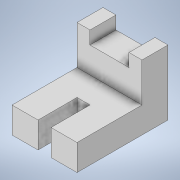
# Autodesk Inventor part: 4.2 Part C
Saved by Autodesk Inventor 2020 (Build 240168000, 168)
## iProperties
Created: 2020-01-07
Part Number: 4.2 Part C
Material: Generic
Document SubType Name: Modeling
Designer: cks4a449
Density: 1 g/cm^3
Appearance: Default
Author: cks4a449
Autodesk Inventor part; units mm, degrees
ref_plane "YZ Plane" through (0, 0, 0) normal (1, 0, 0) x (0, 1, 0)
ref_plane "XZ Plane" through (0, 0, 0) normal (0, 1, 0) x (-1, 0, 0)
ref_plane "XY Plane" through (0, 0, 0) normal (0, 0, 1) x (1, 0, 0)
sketch "Sketch1" plane through (0, 0, 0) normal (0, 0, 1) x (1, 0, 0)
  line L0 (0, 0) -> (88.9, 0)
  line L1 (88.9, 0) -> (88.9, 63.5)
  line L2 (88.9, 63.5) -> (63.5, 63.5)
  line L3 (63.5, 63.5) -> (63.5, 25.4)
  line L4 (63.5, 25.4) -> (0, 25.4)
  line L5 (0, 25.4) -> (0, 0)
  dimension "d0" = 88.9
  dimension "d1" = 63.5
  dimension "d2" = 25.4
  dimension "d3" = 38.1
  constraints: 12 end point, 5 perpendicular, 1 horizontal
  measures "d0" distance of L0.start L0.end
  measures "d1" distance of L0.end L1.end
  measures "d2" distance of L1.end L2.end
  measures "d3" distance of L2.end L3.end
extrude "Extrusion1" add sketch "Sketch1" along normal blind 63.5
sketch "Sketch2" plane through (63.5, 63.5, 0) normal (0, 1, 0) x (1, 0, 0)
  line L0 (25.4, 0) -> (25.4, -63.5) projected
  line L1 (25.4, 0) -> (0, 0)
  line L2 (0, 0) -> (0, -12.7)
  line L3 (0, -12.7) -> (25.4, -12.7)
  line L4 (25.4, -12.7) -> (25.4, 0)
  line L5 (25.4, -12.7) -> (0, -12.7)
  line L6 (0, -12.7) -> (0, -50.8)
  line L7 (0, -50.8) -> (25.4, -50.8)
  line L8 (25.4, -50.8) -> (25.4, -12.7)
  point P0 (-63.5, 0)
  dimension "d6" = 25.4
  dimension "d7" = 12.7
  dimension "d8" = 25.4
  dimension "d9" = 38.1
  constraints: 16 end point, 4 parallel, 2 horizontal, 2 perpendicular
  measures "d6" distance of L3.end L2.end
  measures "d7" distance of L2.end L1.end
  measures "d8" distance of L7.end L6.end
  measures "d9" distance of L6.end L5.end
extrude "Extrusion2" cut sketch "Sketch2" against normal blind 12.7 contours L0 L7 L6 L3
sketch "Sketch3" plane through (0, 0, 0) normal (-1, 0, 0) x (0, 0, 1)
  line L0 (0, 0) -> (0, 63.5) projected
  line L1 (0, 0) -> (25.4, 0)
  line L2 (25.4, 0) -> (25.4, 25.4)
  line L3 (25.4, 25.4) -> (0, 25.4)
  line L4 (0, 25.4) -> (0, 0)
  line L5 (25.4, 25.4) -> (38.1, 25.4)
  line L6 (38.1, 25.4) -> (38.1, 0)
  line L7 (38.1, 0) -> (25.4, 0)
  line L8 (25.4, 0) -> (25.4, 25.4)
  dimension "d12" = 25.4
  dimension "d13" = 25.4
  dimension "d14" = 12.7
  dimension "d15" = 25.4
  constraints: 16 end point, 4 parallel, 2 horizontal, 2 perpendicular
  measures "d12" distance of L3.end L2.end
  measures "d13" distance of L2.end L1.end
  measures "d14" distance of L6.end L7.end
  measures "d15" distance of L5.end L6.end
extrude "Extrusion3" cut sketch "Sketch3" against normal blind 38.1 contours L2 L5 L6 L7
body "Solid1"
